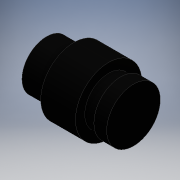
# Autodesk Inventor part: ET21
Saved by Autodesk Inventor 2016 (Build 200138000, 138)
## iProperties
Created: 2016-04-16
Part Number: ET21
Material: Genérico
Document SubType Name: Modeling
Designer: Usuario1
Density: 1 g/cm^3
Appearance: Valor por defecto
Author: Usuario1
Autodesk Inventor part; units mm, degrees
ref_plane "YZ Plane" through (0, 0, 0) normal (1, 0, 0) x (0, 1, 0)
ref_plane "XZ Plane" through (0, 0, 0) normal (0, 1, 0) x (-1, 0, 0)
ref_plane "XY Plane" through (0, 0, 0) normal (0, 0, 1) x (1, 0, 0)
sketch "Boceto1" plane through (0, 0, 0) normal (0, 0, 1) x (1, 0, 0)
  line L0 (0.448, 0.4011) -> (0.448, 0)
  line L1 (0.448, 0) -> (0, 0)
  line L2 (0, 0) -> (0, 0.4011)
  line L3 (1.0145, -0.1407) -> (0.448, -0.1407)
  line L4 (0.448, -0.1407) -> (0.448, 0.4011)
  line L5 (1.2116, 0.4011) -> (1.2116, 0.0112)
  line L6 (1.2116, 0.0112) -> (1.0145, 0.0112)
  line L7 (1.0145, 0.0112) -> (1.0145, 0.4011)
  line L8 (1.4202, 0.4011) -> (1.4202, -0.0366)
  line L9 (1.4202, -0.0366) -> (1.2116, -0.0366)
  line L10 (0, 0.4011) -> (1.4202, 0.4011)
  line L11 (1.2116, -0.0366) -> (1.2116, 0.4011)
  line L12 (1.0145, 0.4011) -> (1.0145, -0.1407)
  constraints: 26 end point, 6 point on line, 1 perpendicular
revolve "Revolución1" add sketch "Boceto1" angle 360 about axis through (0, 0.4011, 0) along (1, 0, 0)
sketch "Boceto2" plane through (0, 0.4011, 0) normal (-1, 0, 0) x (0, 0, 1)
  circle A0 centre (0, 0) radius 0.4011 projected
  line L0 (0.17, 0) -> (0.17, 0.17)
  line L1 (0.17, 0.17) -> (-0.17, 0.17)
  line L2 (-0.17, 0.17) -> (-0.17, -0.17)
  line L3 (-0.17, -0.17) -> (0.17, -0.17)
  line L4 (0.17, -0.17) -> (0.17, 0)
  point P0 (0, -0.4011)
  constraints: 10 end point, 2 perpendicular, 1 vertical alignment
extrude "Extrusión1" cut sketch "Boceto2" against normal blind 0.28 contours L4 L3 L2 L1 L0
